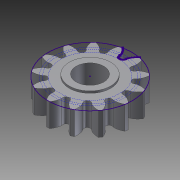
# Autodesk Inventor part: Z13
Saved by Autodesk Inventor 2014 (Build 180170000, 170)
## iProperties
Created: 2013-05-24
Part Number: Z13
Material: Generic
Document SubType Name: Modeling
Designer: hartmann
Density: 1 g/cm^3
Appearance: Default
Mass: 0.0323486 g
Surface Area: 1.05799 cm^2
Volume: 0.0323486 cm^3
Author: hartmann
Autodesk Inventor part; units mm, degrees
ref_plane "YZ Plane" through (0, 0, 0) normal (1, 0, 0) x (0, 1, 0)
ref_plane "XZ Plane" through (0, 0, 0) normal (0, 1, 0) x (-1, 0, 0)
ref_plane "XY Plane" through (0, 0, 0) normal (0, 0, 1) x (1, 0, 0)
sketch "Sketch1" plane through (0, 0, 0) normal (0, 0, 1) x (1, 0, 0)
  spline S0 degree 3 poles (-0.617, 2.9837) (-0.5961, 2.9647) (-0.5543, 2.9267) (-0.4954, 2.8657) (-0.4397, 2.8019) (-0.3878, 2.7349) (-0.3404, 2.6647) (-0.2984, 2.591) (-0.2694, 2.5266) (-0.2505, 2.4733) (-0.2449, 2.4456) (-0.2421, 2.4318) knots 0 0 0 0 0.008469 0.016937 0.025406 0.033874 0.042343 0.05081 0.059276 0.063509 0.06774 0.06774 0.06774 0.06774
  spline S1 degree 3 poles (-0.2421, 2.4318) (-0.2407, 2.4142) (-0.2381, 2.379) (-0.2282, 2.3269) (-0.2111, 2.2767) (-0.1891, 2.2382) (-0.1674, 2.2103) (-0.1481, 2.1921) (-0.1271, 2.176) (-0.1038, 2.1632) (-0.0788, 2.1544) (-0.0443, 2.1464) (0, 2.149) (0.0443, 2.1464) (0.0788, 2.1544) (0.1038, 2.1632) (0.1271, 2.176) (0.1481, 2.1921) (0.1674, 2.2103) (0.1891, 2.2382) (0.2111, 2.2767) (0.2282, 2.3269) (0.2381, 2.379) (0.2407, 2.4142) (0.2421, 2.4318) knots 0 0 0 0 0.005287 0.010573 0.01586 0.021141 0.023788 0.026432 0.029074 0.031719 0.03436 0.037004 0.042291 0.047577 0.050221 0.052863 0.055508 0.058149 0.060794 0.06344 0.068721 0.074009 0.079294 0.084582 0.084582 0.084582 0.084582
  spline S2 degree 3 poles (0.2421, 2.4318) (0.2449, 2.4456) (0.2505, 2.4733) (0.2694, 2.5266) (0.2984, 2.591) (0.3404, 2.6647) (0.3878, 2.7349) (0.4397, 2.8019) (0.4954, 2.8657) (0.5543, 2.9267) (0.5961, 2.9647) (0.617, 2.9837) knots 0 0 0 0 0.004231 0.008465 0.01693 0.025398 0.033866 0.042334 0.050803 0.059272 0.06774 0.06774 0.06774 0.06774
  circle A0 centre (0, 0) radius 2.148 construction
  circle A1 centre (0, 0) radius 2.4432 construction
  circle A2 centre (0, 0) radius 2.6 construction
  circle A3 centre (0, 0) radius 3.0468
  point P0 (-0.555, 2.926)
  point P1 (-0.496, 2.8653)
  point P2 (-0.4403, 2.8014)
  point P3 (-0.3886, 2.7344)
  point P4 (-0.3413, 2.6641)
  point P5 (-0.2996, 2.5904)
  point P6 (-0.2651, 2.5131)
  point P7 (-0.2515, 2.473)
  point P8 (-0.2371, 2.3791)
  point P9 (-0.227, 2.3273)
  point P10 (-0.2095, 2.2773)
  point P11 (-0.1834, 2.2315)
  point P12 (-0.1669, 2.2107)
  point P13 (-0.1478, 2.1925)
  point P14 (-0.1267, 2.1766)
  point P15 (-0.1035, 2.1639)
  point P16 (-0.0787, 2.1549)
  point P17 (-0.0528, 2.1493)
  point P18 (0, 2.148)
  point P19 (0.0528, 2.1493)
  point P20 (0.0787, 2.1549)
  point P21 (0.1035, 2.1639)
  point P22 (0.1267, 2.1766)
  point P23 (0.1478, 2.1925)
  point P24 (0.1669, 2.2107)
  point P25 (0.1834, 2.2315)
  point P26 (0.2095, 2.2773)
  point P27 (0.227, 2.3273)
  point P28 (0.2371, 2.3791)
  point P29 (0.2515, 2.473)
  point P30 (0.2651, 2.5131)
  point P31 (0.2996, 2.5904)
  point P32 (0.3413, 2.6641)
  point P33 (0.3886, 2.7344)
  point P34 (0.4403, 2.8014)
  point P35 (0.496, 2.8653)
  point P36 (0.555, 2.926)
  constraints: 4 centre point, 2 point on circle, 89 other
extrude "Extrusion1" add sketch "Sketch1" against normal blind 1.7
extrude "Extrusion2" cut sketch "Sketch1" against normal through all contours A3 S2 S1 S0 picked at (0.0513, 2.7382)
pattern_circular "Runde Anordnung1" count 13 over 360 about axis through (0, 0, -10) along (0, 0, 1) of "Extrusion2"
sketch "Sketch2" plane through (0, 0, -1.7) normal (0, 0, -1) x (-1, 0, 0)
  arc A0 (-0.617, 2.9837) -> (-0.8402, 2.9286) centre (0, 0) ccw projected
  circle A1 centre (0, 0) radius 1
  dimension "d7" = 2
  constraints: 1 centre point, 1 coincident
  measures "d7" diameter of A1
extrude "Extrusion3" cut sketch "Sketch2" against normal through all
sketch "Sketch3" plane through (0, 0, -1.7) normal (0, 0, -1) x (-1, 0, 0)
  circle A0 centre (0, 0) radius 1 projected
  arc A1 (-0.617, 2.9837) -> (-0.8402, 2.9286) centre (0, 0) ccw projected
  circle A2 centre (0, 0) radius 1.5
  dimension "d10" = 0.5
  constraints: 1 centre point, 1 coincident
  measures "d10" radial gap between concentric circles of A2 A0
extrude "Extrusion4" add sketch "Sketch3" along normal blind 0.15
sketch "Sketch4" plane through (0, 0, 0) normal (0, 0, 1) x (1, 0, 0)
  circle A0 centre (0, 0) radius 1 projected
  circle A1 centre (0, 0) radius 1.5 projected
extrude "Extrusion5" add sketch "Sketch4" along normal blind 0.15
equation "\"Modul\" = 0.4"
equation "\"Druckwinkel\" = 20deg"
equation "\"UnitProfileClearance\" = 0.25"
equation "\"UnitRoundRadius\" = 0.35"
equation "\"Kopfdurchmesser\" = 6.09356"
equation "\"Stammdurchmesser\" = 4.296"
equation "\"Grundkreisdurchmesser\" = 4.8864"
equation "\"Gewindedurchmesser\" = 5.2"
equation "\"Zahnbreite\" = 2"
equation "\"Schrägungswinkel\" = 0"
equation "\"UnitCorrection\" = 0.12"
equation "\"UnitAddendumModification\" = 0.003054"
equation "\"Zahnkreisteilung\" = 1.25664"
equation "\"UnitBacklashShift\" = 0"
equation "\"Gesamtzahnstärke\" = 0.048"
equation "\"Innen\" = 0"
